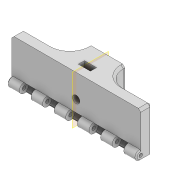
# Autodesk Inventor part: anchor
Saved by Autodesk Inventor 2020 (Build 240168000, 168)
## iProperties
Created: 2020-04-23
Part Number: anchor
Material: Generic
Document SubType Name: Modeling
Designer: Daniel
Density: 1 g/cm^3
Appearance: Default
Mass: 61.348 g
Surface Area: 168.068 cm^2
Volume: 61.348 cm^3
Author: Daniel
Autodesk Inventor part; units mm, degrees
ref_plane "YZ Plane" through (0, 0, 0) normal (1, 0, 0) x (0, 1, 0)
ref_plane "XZ Plane" through (0, 0, 0) normal (0, 1, 0) x (-1, 0, 0)
ref_plane "XY Plane" through (0, 0, 0) normal (0, 0, 1) x (1, 0, 0)
sketch "Sketch1" plane through (0, 0, 0) normal (0, 0, 1) x (1, 0, 0)
  line L0 (0, 0) -> (-31.1, 0)
  line L1 (-31.1, 0) -> (-31.1, 38.1)
  line L2 (-31.1, 38.1) -> (0, 38.1)
  line L3 (0, 38.1) -> (0, 0)
  dimension "d0" = 38.1
  dimension "d1" = 31.1
  constraints: 8 end point, 2 parallel, 1 horizontal, 1 perpendicular
  measures "d0" distance of L0.end L1.end
  measures "d1" distance of L1.end L2.end
extrude "Extrusion1" add sketch "Sketch1" along normal blind 26.3
sketch "Sketch2" plane through (0, 0, 0) normal (0, 0, -1) x (-1, 0, 0)
  circle A0 centre (15.55, 31.55) radius 2.7
  line L0 (0, 38.1) -> (31.1, 38.1) construction
  circle A1 centre (15.55, 6.55) radius 2.7
  line L1 (31.1, 0) -> (0, 0) construction
  line L2 (0, 0) -> (0, 38.1) construction
  line L3 (31.1, 38.1) -> (31.1, 0) construction
  dimension "d4" = 5.4
  dimension "d5" = 6.55
  dimension "d6" = 5.4
  dimension "d7" = 6.55
  dimension "d8" = 15.55
  dimension "d9" = 15.55
  constraints: 2 centre point, 1 vertical alignment
  measures "d4" diameter of A0
  measures "d5" distance from line of L0 A0.centre
  measures "d6" diameter of A1
  measures "d7" distance from line of L1 A1.centre
  measures "d8" distance from line of L2 A0.centre
  measures "d9" distance from line of L3 A0.centre
extrude "Extrusion2" cut sketch "Sketch2" against normal blind 13.3
sketch "Sketch3" plane through (0, 38.1, 0) normal (0, 1, 0) x (0, 0, -1)
  line L0 (-19.3, 20.75) -> (-14, 20.75)
  line L1 (-14, 20.75) -> (-14, 10.35)
  line L2 (-14, 10.35) -> (-19.3, 10.35)
  line L3 (-19.3, 10.35) -> (-19.3, 20.75)
  line L4 (0, 0) -> (-26.3, 0) construction
  line L5 (0, 0) -> (-26.3, 0) construction
  line L6 (-19.3, 15.55) -> (-14, 15.55) construction
  line L7 (0, 31.1) -> (-26.3, 31.1) construction
  line L8 (-26.3, 0) -> (-26.3, 31.1) construction
  dimension "d12" = 5.3
  dimension "d13" = 10.4
  dimension "d43" = 15.55
  dimension "d44" = 15.55
  dimension "d45" = 7
  constraints: 10 end point, 2 midpoint, 2 parallel, 1 horizontal, 1 perpendicular
  measures "d12" distance of L1.end L2.end
  measures "d13" distance of L0.end L1.end
  measures "d43" distance between parallel lines of L4 L6
  measures "d44" distance between parallel lines of L7 L6
  measures "d45" distance between parallel lines of L8 L3
extrude "Extrusion3" cut sketch "Sketch3" against normal blind 27.1
sketch "Sketch4" plane through (0, 0, 26.3) normal (0, 0, 1) x (1, 0, 0)
  line L0 (0, 38.1) -> (-31.1, 38.1) construction
  circle A0 centre (-15.55, 18) radius 3.15
  line L1 (-31.1, 0) -> (0, 0) construction
  line L2 (0, 0) -> (0, 38.1) construction
  line L3 (-31.1, 38.1) -> (-31.1, 0) construction
  dimension "d16" = 6.3
  dimension "d38" = 18
  dimension "d39" = 15.55
  dimension "d40" = 15.55
  constraints: 1 centre point
  measures "d16" diameter of A0
  measures "d38" distance from line of L1 A0.centre
  measures "d39" distance from line of L2 A0.centre
  measures "d40" distance from line of L3 A0.centre
extrude "Extrusion4" cut sketch "Sketch4" against normal through all
sketch "Sketch8" plane through (0, 0, 0) normal (1, 0, 0) x (0, 0, -1)
  point P0 (0, 0)
sketch "Sketch9" plane through (0, 0, 0) normal (1, 0, 0) x (0, 0, -1)
  line L0 (0, 0) -> (-26.3, 0) construction
  line L1 (-26.3, 38.1) -> (-16.3, 38.1)
  line L2 (-16.3, 38.1) -> (-16.3, 0)
  line L3 (-16.3, 0) -> (-26.3, 0)
  line L4 (-26.3, 0) -> (-26.3, 38.1)
  dimension "d32" = 10
  constraints: 8 end point, 2 parallel, 1 horizontal, 1 perpendicular, 1 point on line
  measures "d32" distance between parallel lines of L4 L2
extrude "Extrusion8" add sketch "Sketch9" along normal blind 40
ref_plane "Work Plane2" through (-15.55, 0, 0) normal (1, 0, 0) x (0, 0, -1)
sketch "Sketch5" plane through (-15.55, 0, 0) normal (1, 0, 0) x (0, 0, -1)
  circle A0 centre (-26.3, 4) radius 4
  line L0 (-26.3, 38.1) -> (-26.3, 0) construction
  line L1 (0, 0) -> (-26.3, 0) construction
  point P0 (-18.3, 0)
  dimension "d22" = 8
  constraints: 1 centre point, 1 point on line, 1 tangent
  measures "d22" diameter of A0
extrude "Extrusion5" add sketch "Sketch5" along normal up to surface (55.55 mm away)
mirror "Mirror2" about plane through (-15.55, 0, 0) normal (1, 0, 0) of "Extrusion5", "Extrusion8"
sketch "Sketch6" plane through (40, 0, 0) normal (1, 0, 0) x (0, 0, -1)
  arc A0 (-26.3, 8) -> (-26.3, 0) centre (-26.3, 4) ccw construction
  circle A1 centre (-26.3, 4) radius 1.5
  point P0 (0, 0)
  point P1 (-28.3, 8)
  point P2 (-28.3, 0)
  dimension "d25" = 3
  constraints: 1 centre point, 1 coincident
  measures "d25" diameter of A1
extrude "Extrusion6" cut sketch "Sketch6" against normal through all
sketch "Sketch7" plane through (-15.55, 0, 0) normal (1, 0, 0) x (0, 0, -1)
  arc A0 (-31.3464, 4.4774) -> (-31.3464, 3.5226) centre (-26.3, 4) ccw construction
  circle A1 centre (-26.3, 4) radius 4
  line L0 (-26.3, 4) -> (-24.3, 4)
  line L1 (-24.3, 4) -> (-24.3, -2.0536)
  line L2 (-24.3, -2.0536) -> (-26.3, -2.0536)
  line L3 (-26.3, -2.0536) -> (-26.3, 4)
  circle A2 centre (-26.3, 4) radius 1.5 construction
  point P0 (0, 0)
  point P1 (-24.3, 0.5359)
  point P2 (-26.3, 0)
  dimension "d28" = 8
  dimension "d31" = 2
  constraints: 8 end point, 2 centre point, 2 parallel, 2 point on circle, 1 coincident, 1 concentric, 1 horizontal, 1 perpendicular
  measures "d28" diameter of A1
  measures "d31" distance of L0.start L0.end
extrude "Extrusion7" cut sketch "Sketch7" along normal mid plane 10
pattern_linear "Rectangular Pattern1" count 5 spacing 20 along (1, 0, 0) of "Extrusion7" first direction both ways yes
fillet "Fillet1" radius 15 2 edges at (0, 19.05, 16.3) (-31.1, 19.05, 16.3)
chamfer "Chamfer1" distance 2 angle 45 16 edges at (40, 19.05, 16.3) (-71.1, 19.05, 16.3) (-58.6, 38.1, 16.3) (-35.4934, 38.1, 11.9066) (-31.1, 38.1, 0.65) (4.3934, 38.1, 11.9066) (27.5, 38.1, 16.3) (0, 38.1, 0.65) (4.3934, 0, 11.9066) (0, 0, 0.65) (27.5, 0, 16.3) (-35.4934, 0, 11.9066) (-58.6, 0, 16.3) (-31.1, 0, 0.65) (40, 38.1, 21.3) (-71.1, 38.1, 21.3)
chamfer "Chamfer2" distance 1 angle 45 4 edges at (-71.1, 0, 22.3) (-71.1, 4, 30.3) (40, 0, 22.3) (40, 4, 30.3)
equation "\"d7\" = d5"
equation "\"d8\" = d9"
equation "\"d43\" = d44"
equation "\"d39\" = d40"
body "Solid1"
